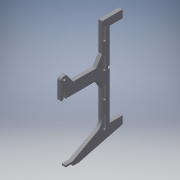
# Autodesk Inventor part: TrayPanelG
Saved by Autodesk Inventor 2017 (Build 210142000, 142)
## iProperties
Created: 2019-06-23
Part Number: TrayPanelG
Material: Generic
Document SubType Name: Modeling
Designer: DDeGo
Density: 1 g/cm^3
Appearance: Default
Author: DDeGo
Autodesk Inventor part; units mm, degrees
ref_plane "YZ Plane" through (0, 0, 0) normal (1, 0, 0) x (0, 1, 0)
ref_plane "XZ Plane" through (0, 0, 0) normal (0, 1, 0) x (-1, 0, 0)
ref_plane "XY Plane" through (0, 0, 0) normal (0, 0, 1) x (1, 0, 0)
sketch "Sketch1" plane through (0, 0, 0) normal (1, 0, 0) x (0, 1, 0)
  line L0 (0, 0) -> (8.6, 0)
  line L1 (8.6, 0) -> (8.6, -2.75)
  line L2 (8.6, -2.75) -> (15.6, -2.75)
  line L3 (15.6, -2.75) -> (66.85, 10.5)
  line L4 (66.85, 10.5) -> (66.85, 19.5)
  line L5 (66.85, 19.5) -> (51.85, 19.5)
  line L6 (51.85, 19.5) -> (51.85, 118.5)
  line L7 (51.85, 118.5) -> (66.85, 118.5)
  line L8 (66.85, 118.5) -> (66.85, 127.5)
  line L9 (42.85, 21) -> (8, 2)
  line L10 (8, 2) -> (0, 2)
  line L11 (0, 2) -> (0, 0)
  line L12 (0, 70) -> (0, 77)
  line L13 (0, 77) -> (-2.75, 77)
  line L14 (-2.75, 77) -> (-2.75, 70)
  line L15 (0, 70) -> (35.85, 70)
  line L16 (35.85, 70) -> (42.85, 59)
  line L17 (42.85, 94) -> (35.85, 83)
  line L18 (35.85, 83) -> (35.85, 70) construction
  line L19 (42.85, 127.5) -> (42.85, 94)
  line L20 (42.85, 59) -> (42.85, 21)
  line L21 (42.85, 127.5) -> (66.85, 127.5)
  line L22 (-1.375, 77) -> (-1.375, 90) construction
  arc A0 (1.866, 92.3443) -> (-5.375, 90) centre (-1.375, 90) ccw
  line L23 (-5.375, 90) -> (-5.375, 70)
  line L24 (1.866, 92.3443) -> (8.625, 83)
  circle A1 centre (-1.375, 90) radius 1.5
  line L25 (35.85, 83) -> (8.625, 83)
  line L26 (-2.75, 70) -> (-5.375, 70)
  dimension "d0" = 2.75
  dimension "d1" = 8.6
  dimension "d2" = 7
  dimension "d3" = 2
  dimension "d4" = 43.25
  dimension "d6" = 15
  dimension "d7" = 99
  dimension "d8" = 9
  dimension "d14" = 19.5
  dimension "d16" = 8
  dimension "d25" = 9
  dimension "d27" = 2.75
  dimension "d29" = 8.6
  dimension "d34" = 7
  dimension "d36" = 9
  dimension "d37" = 9
  dimension "d38" = 7
  dimension "d39" = 35
  dimension "d56" = 8
  dimension "d57" = 3
  dimension "d59" = 10
  dimension "d61" = 38
  dimension "d77" = 13
  dimension "d78" = 75
  dimension "d79" = 13
  dimension "d81" = 2.625
  constraints: 54 end point, 9 perpendicular, 6 horizontal, 2 centre point, 2 coincident, 2 point on circle, 2 point on line, 2 tangent, 2 vertical, 1 collinear, 1 equal length, 1 midpoint, 1 parallel
  measures "d0" distance of L0.end L1.end
  measures "d1" distance of L0.start L0.end
  measures "d2" distance of L1.end L2.end
  measures "d3" distance of L10.end L0.start
  measures "d4" distance between parallel lines of L1 L6
  measures "d6" distance between parallel lines of L6 L4
  measures "d7" distance between parallel lines of L7 L5
  measures "d8" distance of L3.end L4.end
  measures "d14" distance from line of L0.end L5
  measures "d16" distance of L9.end L10.end
  measures "d25" distance of L7.end L8.end
  measures "d27" distance between parallel lines of L12 L14
  measures "d29" distance between parallel lines of L12 L1
  measures "d34" distance of L12.start L12.end
  measures "d36" distance between parallel lines of L6 L20
  measures "d37" distance between parallel lines of L6 L19
  measures "d38" distance between parallel lines of L18 L20
  measures "d39" distance of L17.start L16.end
  measures "d56" diameter of A0
  measures "d57" diameter of A1
  measures "d59" distance from line of L22 L24.end
  measures "d61" distance of L16.end L9.start
  measures "d77" distance between parallel lines of L25 L15
  measures "d78" distance between parallel lines of L10 L13
  measures "d79" distance of L22.start L22.end
  measures "d81" distance of L14.end L23.end
extrude "Extrusion1" add sketch "Sketch1" along normal blind 4.3
sketch "Sketch2" plane through (4.3, 0, 0) normal (1, 0, 0) x (0, 0, -1)
  line L0 (-120.5, 47.225) -> (-105.5, 47.225)
  line L1 (-105.5, 47.225) -> (-105.5, 44.475)
  line L2 (-105.5, 44.475) -> (-120.5, 44.475)
  line L3 (-120.5, 44.475) -> (-120.5, 47.225)
  line L4 (-90.5, 47.225) -> (-75.5, 47.225)
  line L5 (-75.5, 47.225) -> (-75.5, 44.475)
  line L6 (-75.5, 44.475) -> (-90.5, 44.475)
  line L7 (-90.5, 44.475) -> (-90.5, 47.225)
  line L8 (-60.5, 47.225) -> (-45.5, 47.225)
  line L9 (-45.5, 47.225) -> (-45.5, 44.475)
  line L10 (-45.5, 44.475) -> (-60.5, 44.475)
  line L11 (-60.5, 44.475) -> (-60.5, 47.225)
  line L12 (-30.5, 47.225) -> (-15.5, 47.225)
  line L13 (-15.5, 47.225) -> (-15.5, 44.475)
  line L14 (-15.5, 44.475) -> (-30.5, 44.475)
  line L15 (-30.5, 44.475) -> (-30.5, 47.225)
  line L16 (-127.5, 66.85) -> (-127.5, 42.85) projected
  line L17 (-19.5, 51.85) -> (-118.5, 51.85) projected
  line L18 (-127.5, 42.85) -> (-94, 42.85) projected
  line L19 (-105.5, 45.85) -> (-104.169, 45.85) construction
  line L20 (-104.169, 45.85) -> (-104.169, 42.85) construction
  line L21 (-127.5, 42.85) -> (-94, 42.85) projected
  point P0 (0, 0)
  dimension "d43" = 7
  dimension "d44" = 2.75
  dimension "d46" = 15
  dimension "d47" = 30
  dimension "d48" = 30
  dimension "d49" = 15
  dimension "d50" = 15
  dimension "d51" = 15
  dimension "d52" = 30
  dimension "d72" = 3
  constraints: 36 end point, 8 parallel, 5 horizontal, 5 point on line, 4 perpendicular, 2 collinear, 1 midpoint, 1 vertical
  measures "d43" distance between parallel lines of L16 L3
  measures "d44" distance of L2.end L0.start
  measures "d46" distance between parallel lines of L3 L1
  measures "d47" distance between parallel lines of L7 L3
  measures "d48" distance between parallel lines of L7 L11
  measures "d49" distance of L5.end L6.end
  measures "d50" distance of L9.end L10.end
  measures "d51" distance of L13.end L14.end
  measures "d52" distance between parallel lines of L15 L11
  measures "d72" distance of L19.end L20.end
extrude "Extrusion2" cut sketch "Sketch2" against normal blind 10
fillet "Fillet1" radius 10 1 edges at (2.15, 42.85, 21)
sketch "Sketch4" plane through (4.3, 0, 0) normal (1, 0, 0) x (0, 0, -1)
  line L0 (-19.5, 51.85) -> (-118.5, 51.85) projected
  line L1 (-77.875, 51.85) -> (-75.125, 51.85)
  line L2 (-75.125, 51.85) -> (-75.125, 48.85)
  line L3 (-75.125, 48.85) -> (-77.875, 48.85)
  line L4 (-77.875, 48.85) -> (-77.875, 51.85)
  line L5 (-90.5, 47.225) -> (-75.5, 47.225) projected
  line L6 (-77, -2.75) -> (-77, 0) projected
  point P0 (0, 0)
  dimension "d73" = 3
  dimension "d74" = 1.625
  dimension "d82" = 0.875
  dimension "d83" = 2.75
  constraints: 8 end point, 2 parallel, 1 horizontal, 1 perpendicular, 1 point on line
  measures "d73" distance between parallel lines of L0 L3
  measures "d74" distance between parallel lines of L5 L3
  measures "d82" distance between parallel lines of L4 L6
  measures "d83" distance between parallel lines of L4 L2
extrude "Extrusion4" cut sketch "Sketch4" against normal blind 10
body "Solid1"
